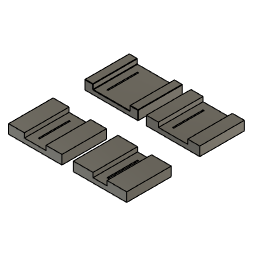
foam_tape_cutting_tool v2 (Autodesk Fusion 360 design; units mm, degrees)
Autodesk Fusion 360 part; units mm, degrees
sketch "24mm_guide" plane through (0, 0, 0) normal (0, 0, 1) x (1, 0, 0)
  line L0 (0, 0) -> (35, 0)
  line L1 (35, 0) -> (35, 29.25)
  line L2 (35, 29.25) -> (0, 29.25)
  line L3 (0, 29.25) -> (0, 0)
  line L4 (5.4, 29.25) -> (5.4, 0)
  line L5 (29.6, 29.25) -> (29.6, 0)
  line L6 (10.025, 24.625) -> (10.775, 24.625)
  line L7 (10.775, 24.625) -> (10.775, 4.625)
  line L8 (10.775, 4.625) -> (10.025, 4.625)
  line L9 (10.025, 4.625) -> (10.025, 24.625)
  dimension "d1" = 24.2
  dimension "d11" = 0.75
  dimension "d12" = 20
  dimension "d13" = 4.625
  dimension "d15" = 4.625
  dimension "d22" = 4.625
  dimension "d32" = 35
  dimension "d34" = 5.4
  dimension "d35" = 5.4
  constraint horizontal L0
  constraint vertical L1
  constraint horizontal L2
  constraint vertical L3
  constraint coincident L0.start L3.end
  constraint coincident L2 L4.start
  constraint perpendicular L2 L4
  constraint coincident L2 L5.start
  constraint perpendicular L2 L5
  constraint horizontal L6
  constraint vertical L7
  constraint horizontal L8
  constraint vertical L9
  measures "d1" distance of L4 L5
  measures "d11" distance of L6.start L6.end
  measures "d12" distance of L6.start L8.end
  measures "d13" distance of L4 L9
  measures "d15" distance of L2 L6
  measures "d22" distance of L0 L8
  measures "d32" distance of L1 L3
  measures "d34" distance of L3 L4
  measures "d35" distance of L1 L5
extrude "Extrude1" add sketch "24mm_guide" along normal blind 6.2 contours L0 L2 L3 L4 | L0 L1 L2 L5 makes body 1 at (0, 9.75, 4.1333) makes body 2 at (29.6, 9.75, 4.1333)
extrude "Extrude2" add sketch "24mm_guide" along normal blind 3 contours L0 L2 L4 L5 bodies 1 2
fillet "Fillet1" radius 0.2 24 edges at (5.4, 14.625, 6.2) (0, 14.625, 6.2) (2.7, 0, 6.2) (2.7, 29.25, 6.2) (5.4, 14.625, 3) (5.4, 0, 4.6) (17.5, 0, 3) (29.6, 0, 4.6) (32.3, 0, 6.2) (35, 0, 3.1) (17.5, 0, 0) (0, 0, 3.1) (17.5, 29.25, 3) (5.4, 29.25, 4.6) (35, 14.625, 6.2) (29.6, 14.625, 6.2) (35, 14.625, 0) (29.6, 29.25, 4.6) (32.3, 29.25, 6.2) (35, 29.25, 3.1) (17.5, 29.25, 0) (0, 29.25, 3.1) (29.6, 14.625, 3) (0, 14.625, 0) on bodies 1
copy_body "Body->Comp1" bodies 1 removing the originals makes body 3 in component "24mm_guide"
sketch "19mm_guide" plane through (0, 0, 0) normal (0, 0, 1) x (1, 0, 0)
  line L0 (-2.525, 0.025) -> (32.475, 0.025)
  line L1 (24.575, 29.275) -> (24.575, 0)
  line L2 (32.475, 0.025) -> (32.475, 29.275)
  line L3 (-2.525, 29.275) -> (-2.525, 0.025)
  line L4 (10, 4.65) -> (10, 24.65)
  line L5 (32.475, 29.275) -> (-2.525, 29.275)
  line L6 (10, 24.65) -> (10.75, 24.65)
  line L7 (5.375, 29.275) -> (5.375, 0)
  line L8 (10.75, 24.65) -> (10.75, 4.65)
  line L9 (10.75, 4.65) -> (10, 4.65)
  point P0 (-2.525, 0.025)
  dimension "d36" = 19.2
  dimension "d37" = 0.75
  dimension "d38" = 20
  dimension "d39" = 4.625
  dimension "d40" = 4.625
  dimension "d41" = 4.625
  dimension "d42" = 35
  dimension "d43" = 7.9
  constraint horizontal L0
  constraint vertical L2
  constraint horizontal L5
  constraint vertical L3
  constraint coincident P0 L0.start
  constraint coincident L7.start L5
  constraint perpendicular L5 L7
  constraint coincident L1.start L5
  constraint perpendicular L1 L5
  constraint horizontal L6
  constraint vertical L8
  constraint horizontal L9
  constraint vertical L4
  measures "d36" distance of L1 L7
  measures "d37" distance of L6.end L4.end
  measures "d38" distance of L4.end L4.start
  measures "d39" distance of L4 L7
  measures "d40" distance of L5 L6
  measures "d41" distance of L0 L9
  measures "d42" distance of L2 L3
  measures "d43" distance of L3 L7
extrude "Extrude3" add sketch "19mm_guide" along normal blind 6 separate body contours L0 L3 L5 L7 | L0 L1 L2 L5 makes body 4 at (0.1083, 19.525, 0) makes body 5 at (27.2083, 19.525, 0)
extrude "Extrude4" add sketch "19mm_guide" along normal blind 3 contours L0 L1 L5 L7 bodies 4 5
copy_body "Body->Comp2" bodies 4 removing the originals makes body 6 in component "19mm_guide"
sketch "14mm_guide" plane through (0, 0, 0) normal (0, 0, 1) x (1, 0, 0)
  line L0 (30.025, 29.275) -> (-4.975, 29.275)
  line L1 (10.8, 24.65) -> (10.8, 4.65)
  line L2 (30.025, 0.025) -> (30.025, 29.275)
  line L3 (10.05, 4.65) -> (10.05, 24.65)
  line L4 (10.8, 4.65) -> (10.05, 4.65)
  line L5 (19.625, 29.275) -> (19.625, 0)
  line L6 (5.425, 29.275) -> (5.425, 0)
  line L7 (-4.975, 0.025) -> (30.025, 0.025)
  line L8 (10.05, 24.65) -> (10.8, 24.65)
  line L9 (-4.975, 29.275) -> (-4.975, 0.025)
  point P0 (-4.975, 0.025)
  dimension "d49" = 14.2
  dimension "d50" = 0.75
  dimension "d51" = 20
  dimension "d52" = 4.625
  dimension "d53" = 4.625
  dimension "d54" = 4.625
  dimension "d55" = 35
  dimension "d56" = 10.4
  constraint horizontal L7
  constraint vertical L2
  constraint horizontal L0
  constraint vertical L9
  constraint coincident P0 L7.start
  constraint coincident L6.start L0
  constraint perpendicular L0 L6
  constraint coincident L5.start L0
  constraint perpendicular L0 L5
  constraint horizontal L8
  constraint vertical L1
  constraint horizontal L4
  constraint vertical L3
  measures "d49" distance of L5 L6
  measures "d50" distance of L3.end L1.start
  measures "d51" distance of L3.start L3.end
  measures "d52" distance of L3 L6
  measures "d53" distance of L0 L8
  measures "d54" distance of L4 L7
  measures "d55" distance of L2 L9
  measures "d56" distance of L6 L9
extrude "Extrude5" add sketch "14mm_guide" along normal blind 6 separate body contours L0 L2 L5 L7 | L0 L6 L7 L9 makes body 7 at (-1.5083, 19.525, 0) makes body 8 at (23.0917, 19.525, 0)
extrude "Extrude6" add sketch "14mm_guide" along normal blind 3 contours L0 L5 L6 L7 bodies 7 8
copy_body "Body->Comp3" bodies 7 removing the originals makes body 9 in component "14mm_guide"
sketch "9mm_guide" plane through (0, 0, 0) normal (0, 0, 1) x (1, 0, 0)
  line L0 (14.625, 29.275) -> (14.625, 0)
  line L1 (-7.475, 0.025) -> (27.525, 0.025)
  line L2 (10.8, 24.65) -> (10.8, 4.65)
  line L3 (10.8, 4.65) -> (10.05, 4.65)
  line L4 (27.525, 0.025) -> (27.525, 29.275)
  line L5 (27.525, 29.275) -> (-7.475, 29.275)
  line L6 (10.05, 24.65) -> (10.8, 24.65)
  line L7 (5.425, 29.275) -> (5.425, 0)
  line L8 (10.05, 4.65) -> (10.05, 24.65)
  line L9 (-7.475, 29.275) -> (-7.475, 0.025)
  point P0 (-7.475, 0.025)
  dimension "d63" = 9.2
  dimension "d64" = 0.75
  dimension "d65" = 20
  dimension "d66" = 4.625
  dimension "d67" = 4.625
  dimension "d68" = 4.625
  dimension "d69" = 35
  dimension "d70" = 12.9
  constraint horizontal L1
  constraint vertical L4
  constraint horizontal L5
  constraint vertical L9
  constraint coincident P0 L1.start
  constraint coincident L7.start L5
  constraint perpendicular L5 L7
  constraint coincident L0.start L5
  constraint perpendicular L0 L5
  constraint horizontal L6
  constraint vertical L2
  constraint horizontal L3
  constraint vertical L8
  measures "d63" distance of L0 L7
  measures "d64" distance of L6.start L2.start
  measures "d65" distance of L3.end L6.start
  measures "d66" distance of L7 L8
  measures "d67" distance of L5 L6
  measures "d68" distance of L1 L3
  measures "d69" distance of L4 L9
  measures "d70" distance of L7 L9
extrude "Extrude7" add sketch "9mm_guide" along normal blind 6 separate body contours L0 L1 L4 L5 | L1 L5 L7 L9 makes body 10 at (-3.175, 19.525, 0) makes body 11 at (18.925, 19.525, 0)
extrude "Extrude8" add sketch "9mm_guide" along normal blind 3 contours L0 L1 L5 L7 bodies 10 11
copy_body "Body->Comp4" bodies 10 removing the originals makes body 12 in component "9mm_guide"
component "24mm_guide" placed x (1, 0, 0) y (0, 1, 0) z (0, 0, 1) at (0, 0, 0)
component "19mm_guide" placed x (1, 0, 0) y (0, 1, 0) z (0, 0, 1) at (43, 0, 0)
component "14mm_guide" placed x (1, 0, 0) y (0, 1, 0) z (0, 0, 1) at (95, 0, 0)
component "9mm_guide" placed x (1, 0, 0) y (0, 1, 0) z (0, 0, 1) at (0, 0, 0)
equation "d1 = tape_24 + tolerance"
equation "tape_24 = 24 mm"
equation "tolerance = 0.2 mm"
equation "tape_thickness = 3 mm"
equation "bumpers = 5 mm"
equation "roof_thickness = 3 mm"
equation "slot_width = 0.55 mm"
equation "slot_lenght = 20 mm"
equation "d11 = slot_width + tolerance"
equation "d12 = slot_lenght"
equation "d13 = strip_width - ( ( slot_width + tolerance ) / 2 )"
equation "strip_width = 5 mm"
equation "d15 = d13"
equation "d16 = roof_thickness + tape_thickness + tolerance"
equation "d18 = roof_thickness"
equation "d22 = d15"
equation "d32 = body_width"
equation "body_width = 35 mm"
equation "d34 = ( body_width - ( tape_24 + tolerance ) ) / 2"
equation "d36 = tape_19mm + tolerance"
equation "d37 = slot_width + tolerance"
equation "d38 = slot_lenght"
equation "d39 = strip_width - ( ( slot_width + tolerance ) / 2 )"
equation "d40 = d13"
equation "d41 = d15"
equation "d42 = body_width"
equation "d43 = ( body_width - ( tape_19mm + tolerance ) ) / 2"
equation "tape_19mm = 19 mm"
equation "d45 = roof_thickness + tape_thickness"
equation "d47 = roof_thickness"
equation "d49 = tape_14 + tolerance"
equation "d50 = slot_width + tolerance"
equation "d51 = slot_lenght"
equation "d52 = strip_width - ( ( slot_width + tolerance ) / 2 )"
equation "d53 = d13"
equation "d54 = d15"
equation "d55 = body_width"
equation "d56 = ( body_width - ( tape_14 + tolerance ) ) / 2"
equation "tape_14 = 14 mm"
equation "d58 = roof_thickness + tape_thickness"
equation "d60 = roof_thickness"
equation "tape_9 = 9 mm"
equation "d63 = tape_9 + tolerance"
equation "d64 = slot_width + tolerance"
equation "d65 = slot_lenght"
equation "d66 = strip_width - ( ( slot_width + tolerance ) / 2 )"
equation "d67 = d13"
equation "d68 = d15"
equation "d69 = body_width"
equation "d70 = ( body_width - ( tape_9 + tolerance ) ) / 2"
equation "d71 = roof_thickness + tape_thickness"
equation "d73 = roof_thickness"
